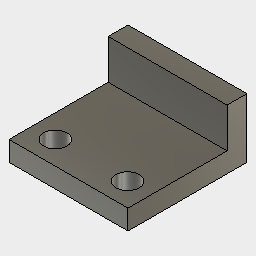
bart pro xl y clip v2 (Autodesk Fusion 360 design; units mm, degrees)
Autodesk Fusion 360 part; units mm, degrees
sketch "Sketch1" plane through (0, 0, 0) normal (0, 0, 1) x (1, 0, 0)
  line L0 (0, 0) -> (18, 0)
  line L1 (18, 0) -> (18, 18)
  line L2 (18, 18) -> (0, 18)
  line L3 (0, 18) -> (0, 0)
  dimension "d1" = 18
  dimension "d2" = 18
  constraint horizontal L0
  constraint vertical L1
  constraint horizontal L2
  constraint vertical L3
extrude "Extrude1" add sketch "Sketch1" along normal blind 3
sketch "Sketch2" plane through (0, 0, 3) normal (0, 0, 1) x (-1, 0, 0)
  line L0 (0, -18) -> (0, 0)
  line L1 (0, 0) -> (-18, 0)
  line L2 (-18, 0) -> (-18, -18)
  line L3 (-18, -18) -> (0, -18)
  line L4 (0, -18) -> (-18, -18)
  line L5 (-18, -18) -> (-18, -15)
  line L6 (-18, -15) -> (0, -15)
  line L7 (0, -15) -> (0, -18)
  dimension "d5" = 3
  constraint vertical L5
  constraint horizontal L6
  constraint vertical L7
extrude "Extrude2" add sketch "Sketch2" along normal blind 6 contours L0 L2 L3 L4 L5 L6 L7
sketch "Sketch3" plane through (0, 0, 0) normal (0, 0, -1) x (1, 0, 0)
  line L0 (0, 0) -> (0, -18)
  line L1 (0, -18) -> (18, -18)
  line L2 (18, -18) -> (18, 0)
  line L3 (18, 0) -> (0, 0)
  line L4 (9, 0) -> (9, -21.7398) construction
  line L5 (3.5, -11.5053) -> (3.5, -21.539) construction
  line L6 (25, 0) -> (25, -0.5298)
  line L7 (25, -0.5298) -> (25, -10.5298) construction
  line L8 (25, -10.5298) -> (24.4826, -10.5298)
  line L9 (25, -10.5298) -> (25, -14.5298) construction
  line L10 (18, -18) -> (0, -18)
  line L11 (14.4421, -18) -> (14.4421, -12) construction
  line L12 (3.5, -11.5053) -> (3.5, 2) construction
  line L13 (14.4421, -12) -> (14.4421, 2.6036) construction
  line L14 (22, 0) -> (22, -3.5) construction
  line L15 (22, -3.5) -> (21, -3.5) construction
  line L16 (21, -3.5) -> (-2, -3.5) construction
  dimension "d11" = 13.5053
  dimension "d12" = 3.5
  constraint midpoint L3
  constraint perpendicular L1 L4
  constraint perpendicular L3 L6
  constraint perpendicular L7 L8
  constraint coincident L1
  constraint perpendicular L3 L12
  constraint perpendicular L14 L15
  constraint perpendicular L0 L16
  constraint coincident L16
  constraint coincident L13
  constraint coincident L12
hole "Hole1" at (3.5, 3.5, 0) direction (0, 0, 1) diameter 3.5 end through all
hole "Hole2" at (14.4421, 3.5, 0) direction (0, 0, 1) diameter 3.5 end through all
